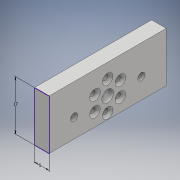
# Autodesk Inventor part: mounting
Saved by Autodesk Inventor 2018 (Build 220112000, 112)
## iProperties
Created: 2017-09-20
Part Number: mounting
Material: Generic
Document SubType Name: Modeling
Designer: Yikealo
Density: 1 g/cm^3
Appearance: Default
Author: Yikealo
Autodesk Inventor part; units mm, degrees
ref_plane "YZ Plane" through (0, 0, 0) normal (1, 0, 0) x (0, 1, 0)
ref_plane "XZ Plane" through (0, 0, 0) normal (0, 1, 0) x (-1, 0, 0)
sketch "Sketch1" plane through (0, 0, 0) normal (0, 1, 0) x (-1, 0, 0)
  line L0 (0, 0) -> (5, 0)
  line L1 (5, 0) -> (5, -17)
  line L2 (5, -17) -> (0, -17)
  line L3 (0, -17) -> (0, 0)
  dimension "d0" = 5
  dimension "d1" = 17
  constraints: 8 end point, 2 parallel, 1 horizontal, 1 perpendicular
  measures "d0" distance of L1.end L2.end
  measures "d1" distance of L0.end L1.end
extrude "Extrusion1" add sketch "Sketch1" along normal blind 40
sketch "Sketch2" plane through (-5, 0, -17) normal (-1, 0, 0) x (0, 0, 1)
  line L0 (17, 0) -> (17, 40) projected
  line L1 (17, 20) -> (-0.1378, 20)
  circle A0 centre (7, 20) radius 2
  line L2 (0, 0) -> (17, 0) projected
  line L3 (6.5, -6.3182) -> (6.5, 42.5723) construction
  line L4 (0, 0) -> (0, 40) projected
  circle A1 centre (6.5, 8.5109) radius 0.5
  circle A2 centre (7, 31.5) radius 0.5
  dimension "d4" = 4
  dimension "d7" = 6.5
  dimension "d9" = 11.5
  dimension "d10" = 1
  dimension "d11" = 1
  dimension "d12" = 0.5
  dimension "d13" = 11.5
  dimension "d105" = 7
  constraints: 4 end point, 3 centre point, 2 point on line, 1 horizontal, 1 midpoint, 1 vertical
  measures "d4" diameter of A0
  measures "d7" distance between parallel lines of L3 L4
  measures "d9" distance of A1.centre A0.centre
  measures "d10" diameter of A1
  measures "d11" diameter of A2
  measures "d12" distance from line of A2.centre L3
  measures "d13" distance of A0.centre A2.centre
  measures "d105" distance from line of A0.centre L4
extrude "Extrusion2" cut sketch "Sketch2" against normal through all contours A0 L1 | L1 A0 | A1 | A2
hole "Hole1" at (-5, 8.5109, -10.5) direction (1, 0, 0) diameter 2.4 end through all clearance for "Flat Head Machine Screw" size "M2" standard "Ansi Metric M Profile"
hole "Hole2" at (-5, 31.5, -10) direction (1, 0, 0) diameter 2.4 end through all clearance for "Flat Head Machine Screw" size "M2" standard "Ansi Metric M Profile"
sketch "Sketch3" plane through (-5, 0, -17) normal (-1, 0, 0) x (0, 0, 1)
  circle A0 centre (7, 20) radius 2 projected
  circle A1 centre (7, 20) radius 5 construction
  line L0 (7, 20) -> (16.0941, 20)
  circle A2 centre (12, 20) radius 0.5
  circle A3 centre (9.5, 24.3301) radius 0.5
  circle A4 centre (4.5, 24.3301) radius 0.5
  circle A5 centre (2, 20) radius 0.5
  circle A6 centre (4.5, 15.6699) radius 0.5
  circle A7 centre (9.5, 15.6699) radius 0.5
  point P0 (17, 0)
  dimension "d32" = 10
  dimension "d33" = 1
  dimension "d36" = 360
  constraints: 6 centre point, 2 end point, 1 coincident, 1 horizontal, 1 horizontal alignment, 1 point on line, 15 other
  measures "d33" diameter of A2
extrude "Extrusion3" cut sketch "Sketch3" against normal through all contours A2 L0 | L0 A2 | A3 | A4 | A5 | A6 | A7
hole "Hole3" at (-5, 20, -5) direction (1, 0, 0) diameter 1.8 end through all countersink diameter 3.6 countersink angle 90 clearance for "Countersunk Flat Head Screw DIN EN ISO 2009" size "M1.6" standard "DIN"
hole "Hole4" at (-5, 15.6699, -7.5) direction (1, 0, 0) diameter 1.8 end through all countersink diameter 3.6 countersink angle 90 clearance for "Countersunk Flat Head Screw DIN EN ISO 2009" size "M1.6" standard "DIN"
hole "Hole5" at (-5, 15.6699, -12.5) direction (1, 0, 0) diameter 1.8 end through all countersink diameter 3.6 countersink angle 90 clearance for "Countersunk Flat Head Screw DIN EN ISO 2009" size "M1.6" standard "DIN"
hole "Hole6" at (-5, 20, -15) direction (1, 0, 0) diameter 1.8 end through all countersink diameter 3.6 countersink angle 90 clearance for "Countersunk Flat Head Screw DIN EN ISO 2009" size "M1.6" standard "DIN"
hole "Hole7" at (-5, 24.3301, -12.5) direction (1, 0, 0) diameter 1.8 end through all countersink diameter 3.6 countersink angle 90 clearance for "Countersunk Flat Head Screw DIN EN ISO 2009" size "M1.6" standard "DIN"
hole "Hole8" at (-5, 24.3301, -7.5) direction (1, 0, 0) diameter 1.8 end through all countersink diameter 3.6 countersink angle 90 clearance for "Countersunk Flat Head Screw DIN EN ISO 2009" size "M1.6" standard "DIN"
ref_plane "Work Plane1" through (-2.5, 0, -17) normal (-1, 0, 0) x (0, 0, 1)
mirror "Mirror1" about plane through (-2.5, 0, -17) normal (-1, 0, 0) of "Hole6", "Hole5", "Hole4", "Hole3", "Hole8", "Hole7"
sketch "Sketch6" plane through (-5, 0, -17) normal (-1, 0, 0) x (0, 0, 1)
  circle A0 centre (7, 20) radius 2 projected
  circle A1 centre (7, 20) radius 9
  point P0 (17, 0)
  dimension "d102" = 18
  constraints: 1 centre point, 1 coincident
  measures "d102" diameter of A1
extrude "Extrusion6" cut sketch "Sketch6" against normal blind 2.5
body "Solid1"
